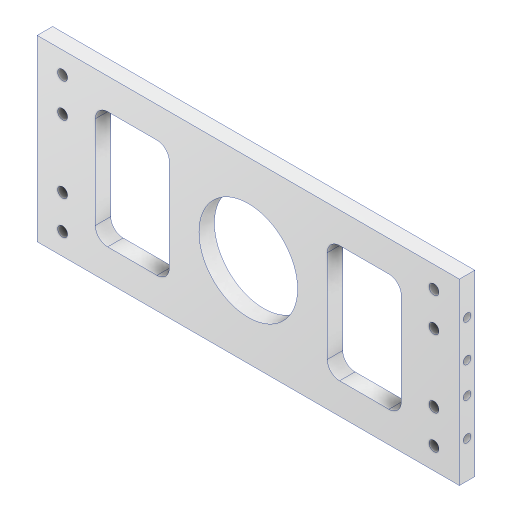
# Autodesk Inventor part: 조인트3_박스아랫판_6T
Saved by Autodesk Inventor 2023.2 (Build 272271000, 271)
## iProperties
Created: 2022-01-24
Part Number: 조인트3_박스아랫판_6T
Material: 알루미늄 6061
Document SubType Name: Modeling
Designer: BAEK
Density: 2.7 g/cm^3
Appearance: 알루미늄 - 평지
Mass: 60.1981 g
Surface Area: 152.316 cm^2
Volume: 22.2956 cm^3
Author: BAEK
Autodesk Inventor part; units mm, degrees
ref_plane "YZ Plane" through (0, 0, 0) normal (1, 0, 0) x (0, 1, 0)
ref_plane "XZ Plane" through (0, 0, 0) normal (0, 1, 0) x (-1, 0, 0)
ref_plane "XY Plane" through (0, 0, 0) normal (0, 0, 1) x (1, 0, 0)
sketch "스케치1" plane through (0, 0, 0) normal (0, 0, 1) x (1, 0, 0)
  line L0 (0, 0) -> (0, 58)
  line L1 (0, 58) -> (129.5, 58)
  line L2 (31.75, 58) -> (31.75, 0) construction
  circle A0 centre (31.75, 51) radius 1.6
  circle A1 centre (31.75, 40) radius 1.6
  circle A2 centre (31.75, 18) radius 1.6
  circle A3 centre (31.75, 7) radius 1.6
  line L3 (64.75, 58) -> (64.75, 0) construction
  circle A4 centre (97.75, 51) radius 1.6
  circle A5 centre (97.75, 40) radius 1.6
  circle A6 centre (97.75, 18) radius 1.6
  circle A7 centre (97.75, 7) radius 1.6
  line L4 (129.5, 58) -> (129.5, 0)
  line L5 (129.5, 0) -> (0, 0)
  circle A8 centre (64.75, 29) radius 10
  dimension "d0" = 58
  dimension "d1" = 129.5
  dimension "d3" = 3.2
  dimension "d4" = 3.2
  dimension "d5" = 3.2
  dimension "d6" = 3.2
  dimension "d7" = 7
  dimension "d8" = 11
  dimension "d9" = 7
  dimension "d10" = 11
  dimension "d13" = 66
  dimension "d14" = 20
  constraints: 12 end point, 9 centre point, 5 point on line, 4 symmetric about line, 4 vertical, 2 midpoint, 2 perpendicular, 4 other
  measures "d0" distance of L0.start L0.end
  measures "d1" distance of L0.end L1.end
  measures "d3" diameter of A0
  measures "d4" diameter of A1
  measures "d5" diameter of A2
  measures "d6" diameter of A3
  measures "d7" distance of L2.start A0.centre
  measures "d8" distance of A0.centre A1.centre
  measures "d9" distance of L2.end A3.centre
  measures "d10" distance of A2.centre A3.centre
  measures "d13" distance of A4.centre A0.centre
  measures "d14" diameter of A8
extrude "돌출1" add sketch "스케치1" along normal blind 4 contours L0 L1 L4 L5 | A8
extrude "돌출2" cut sketch "스케치1" along normal blind 4 contours A8
sketch "스케치2" plane through (0, 0, 4) normal (0, 0, 1) x (1, 0, 0)
  circle A0 centre (64.75, 29) radius 10 projected
  line L0 (0, 58) -> (0, 0) projected
  line L1 (0, 0) -> (129.5, 0) projected
  line L2 (129.5, 0) -> (129.5, 58) projected
  line L3 (129.5, 58) -> (0, 58) projected
  circle A1 centre (97.75, 7) radius 1.6 projected
  circle A2 centre (97.75, 18) radius 1.6 projected
  circle A3 centre (97.75, 40) radius 1.6 projected
  circle A4 centre (97.75, 51) radius 1.6 projected
  circle A5 centre (31.75, 7) radius 1.6 projected
  circle A6 centre (31.75, 18) radius 1.6 projected
  circle A7 centre (31.75, 40) radius 1.6 projected
  circle A8 centre (31.75, 51) radius 1.6 projected
  line L4 (41.75, 51) -> (87.75, 51)
  line L5 (89.75, 49) -> (89.75, 48)
  line L6 (87.75, 46) -> (41.75, 46)
  line L7 (39.75, 48) -> (39.75, 49)
  line L8 (0, 58) -> (0, 0) projected
  line L9 (0, 29) -> (129.5, 29) construction
  line L10 (41.75, 7) -> (87.75, 7)
  line L11 (89.75, 9) -> (89.75, 10)
  line L12 (87.75, 12) -> (41.75, 12)
  line L13 (39.75, 10) -> (39.75, 9)
  arc A9 (41.75, 51) -> (39.75, 49) centre (41.75, 49) ccw
  arc A10 (39.75, 48) -> (41.75, 46) centre (41.75, 48) ccw
  arc A11 (89.75, 49) -> (87.75, 51) centre (87.75, 49) ccw
  arc A12 (87.75, 46) -> (89.75, 48) centre (87.75, 48) ccw
  arc A13 (89.75, 10) -> (87.75, 12) centre (87.75, 10) ccw
  arc A14 (87.75, 7) -> (89.75, 9) centre (87.75, 9) ccw
  arc A15 (39.75, 9) -> (41.75, 7) centre (41.75, 9) ccw
  arc A16 (41.75, 12) -> (39.75, 10) centre (41.75, 10) ccw
  point P0 (39.75, 51)
  point P1 (89.75, 51)
  point P2 (89.75, 46)
  point P3 (39.75, 46)
  point P4 (39.75, 7)
  point P5 (89.75, 7)
  point P6 (89.75, 12)
  point P7 (39.75, 12)
  dimension "d17" = 50
  dimension "d18" = 5
  dimension "d19" = 8
  dimension "d22" = 2
  constraints: 18 end point, 16 point on circle, 16 point on line, 16 tangent, 8 centre point, 7 equal radius, 4 symmetric about line, 2 midpoint, 2 perpendicular, 1 horizontal, 1 vertical
  measures "d17" distance of point (39.75, 51) point (89.75, 51)
  measures "d18" distance of point (89.75, 51) point (89.75, 46)
  measures "d19" distance from line of A8.centre L7
  measures "d22" radius of A9
extrude "돌출3" cut sketch "스케치2" against normal blind 4 contours L4 A11 L5 A12 L6 A10 L7 A9 | A15 L13 A16 L12 A13 L11 A14 L10
sketch "스케치3" plane through (0, 0, 4) normal (0, 0, 1) x (1, 0, 0)
  line L0 (41.75, 12) -> (87.75, 12) projected
  arc A0 (89.75, 10) -> (87.75, 12) centre (87.75, 10) ccw projected
  line L1 (89.75, 10) -> (89.75, 9) projected
  arc A1 (87.75, 7) -> (89.75, 9) centre (87.75, 9) ccw projected
  line L2 (87.75, 7) -> (41.75, 7) projected
  arc A2 (39.75, 9) -> (41.75, 7) centre (41.75, 9) ccw projected
  line L3 (39.75, 9) -> (39.75, 10) projected
  arc A3 (41.75, 12) -> (39.75, 10) centre (41.75, 10) ccw projected
  arc A4 (87.75, 46) -> (89.75, 48) centre (87.75, 48) ccw projected
  line L4 (87.75, 46) -> (41.75, 46) projected
  arc A5 (39.75, 48) -> (41.75, 46) centre (41.75, 48) ccw projected
  line L5 (39.75, 48) -> (39.75, 49) projected
  arc A6 (41.75, 51) -> (39.75, 49) centre (41.75, 49) ccw projected
  line L6 (41.75, 51) -> (87.75, 51) projected
  arc A7 (89.75, 49) -> (87.75, 51) centre (87.75, 49) ccw projected
  line L7 (89.75, 49) -> (89.75, 48) projected
  circle A8 centre (64.75, 29) radius 10 projected
  line L8 (129.5, 0) -> (129.5, 58) projected
  line L9 (129.5, 58) -> (0, 58) projected
  line L10 (0, 58) -> (0, 0) projected
  line L11 (0, 0) -> (129.5, 0) projected
  circle A9 centre (97.75, 7) radius 1.6 projected
  circle A10 centre (97.75, 18) radius 1.6 projected
  circle A11 centre (97.75, 40) radius 1.6 projected
  circle A12 centre (97.75, 51) radius 1.6 projected
  circle A13 centre (31.75, 7) radius 1.6 projected
  circle A14 centre (31.75, 18) radius 1.6 projected
  circle A15 centre (31.75, 40) radius 1.6 projected
  circle A16 centre (31.75, 51) radius 1.6 projected
  line L12 (129.5, 58) -> (0, 58) projected
  line L13 (4.5, 58) -> (4.5, 0)
  line L14 (0, 0) -> (129.5, 0) projected
  circle A17 centre (4.5, 51) radius 1.6
  circle A18 centre (4.5, 40) radius 1.6
  circle A19 centre (4.5, 18) radius 1.6
  circle A20 centre (4.5, 7) radius 1.6
  line L15 (64.75, 58) -> (64.75, 0)
  circle A21 centre (125, 51) radius 1.6
  circle A22 centre (125, 40) radius 1.6
  circle A23 centre (125, 18) radius 1.6
  circle A24 centre (125, 7) radius 1.6
  dimension "d23" = 4.5
  dimension "d24" = 3.2
  dimension "d25" = 3.2
  dimension "d26" = 3.2
  dimension "d27" = 3.2
  constraints: 8 centre point, 6 point on line, 4 end point, 4 symmetric about line, 2 midpoint, 1 perpendicular, 4 other
  measures "d23" distance between parallel lines of L10 L13
  measures "d24" diameter of A17
  measures "d25" diameter of A18
  measures "d26" diameter of A19
  measures "d27" diameter of A20
extrude "돌출4" cut sketch "스케치3" against normal blind 4 contours A20 L13 | L13 A20 | A19 L13 | L13 A19 | A17 L13 | L13 A17 | A18 L13 | L13 A18 | A21 | A22 | A23 | A24
sketch "스케치5" plane through (0, 0, 4) normal (0, 0, 1) x (1, 0, 0)
  circle A0 centre (4.5, 18) radius 1.6 projected
  circle A1 centre (125, 18) radius 1.6 projected
  circle A2 centre (125, 40) radius 1.6 projected
  circle A3 centre (4.5, 40) radius 1.6 projected
  circle A4 centre (4.5, 7) radius 1.6 projected
  circle A5 centre (125, 7) radius 1.6 projected
  circle A6 centre (125, 51) radius 1.6 projected
  circle A7 centre (4.5, 51) radius 1.6 projected
  line L0 (41.75, 12) -> (87.75, 12) projected
  arc A8 (89.75, 10) -> (87.75, 12) centre (87.75, 10) ccw projected
  line L1 (89.75, 10) -> (89.75, 9) projected
  arc A9 (87.75, 7) -> (89.75, 9) centre (87.75, 9) ccw projected
  line L2 (87.75, 7) -> (41.75, 7) projected
  arc A10 (39.75, 9) -> (41.75, 7) centre (41.75, 9) ccw projected
  line L3 (39.75, 9) -> (39.75, 10) projected
  arc A11 (41.75, 12) -> (39.75, 10) centre (41.75, 10) ccw projected
  arc A12 (87.75, 46) -> (89.75, 48) centre (87.75, 48) ccw projected
  line L4 (87.75, 46) -> (41.75, 46) projected
  arc A13 (39.75, 48) -> (41.75, 46) centre (41.75, 48) ccw projected
  line L5 (39.75, 48) -> (39.75, 49) projected
  arc A14 (41.75, 51) -> (39.75, 49) centre (41.75, 49) ccw projected
  line L6 (41.75, 51) -> (87.75, 51) projected
  arc A15 (89.75, 49) -> (87.75, 51) centre (87.75, 49) ccw projected
  line L7 (89.75, 49) -> (89.75, 48) projected
  circle A16 centre (64.75, 29) radius 10 projected
  line L8 (129.5, 0) -> (129.5, 58) projected
  line L9 (129.5, 58) -> (0, 58) projected
  line L10 (0, 58) -> (0, 0) projected
  line L11 (0, 0) -> (129.5, 0) projected
  circle A17 centre (97.75, 7) radius 1.6 projected
  circle A18 centre (97.75, 51) radius 1.6 projected
  circle A19 centre (31.75, 7) radius 1.6 projected
  circle A20 centre (31.75, 51) radius 1.6 projected
  line L12 (129.5, 58) -> (0, 58) projected
  line L13 (64.75, 58) -> (-3.75, 58)
  line L14 (129.5, 58) -> (0, 58) projected
  line L15 (64.75, 58) -> (133.25, 58)
  line L16 (-3.75, 58) -> (-3.75, 0)
  line L17 (0, 0) -> (129.5, 0) projected
  line L18 (-3.75, 0) -> (0, 0)
  line L19 (133.25, 58) -> (133.25, 0)
  line L20 (133.25, 0) -> (129.5, 0)
  dimension "d36" = 68.5
  dimension "d37" = 68.5
  constraints: 12 end point, 2 perpendicular, 2 vertical, 1 horizontal, 1 midpoint, 1 point on line
  measures "d36" distance of L13.start L13.end
  measures "d37" distance of L13.start L15.end
extrude "돌출6" add sketch "스케치5" against normal up to surface (4 mm away) contours L8 L15 L19 L20 | L18 L16 L13 L10
sketch "스케치6" plane through (0, 0, 4) normal (0, 0, 1) x (1, 0, 0)
  circle A0 centre (4.5, 18) radius 1.6 projected
  circle A1 centre (125, 18) radius 1.6 projected
  circle A2 centre (125, 40) radius 1.6 projected
  circle A3 centre (4.5, 40) radius 1.6 projected
  circle A4 centre (4.5, 7) radius 1.6 projected
  circle A5 centre (125, 7) radius 1.6 projected
  circle A6 centre (125, 51) radius 1.6 projected
  circle A7 centre (4.5, 51) radius 1.6 projected
  line L0 (41.75, 12) -> (87.75, 12) projected
  arc A8 (89.75, 10) -> (87.75, 12) centre (87.75, 10) ccw projected
  line L1 (89.75, 10) -> (89.75, 9) projected
  arc A9 (87.75, 7) -> (89.75, 9) centre (87.75, 9) ccw projected
  line L2 (87.75, 7) -> (41.75, 7) projected
  arc A10 (39.75, 9) -> (41.75, 7) centre (41.75, 9) ccw projected
  line L3 (39.75, 9) -> (39.75, 10) projected
  arc A11 (41.75, 12) -> (39.75, 10) centre (41.75, 10) ccw projected
  arc A12 (87.75, 46) -> (89.75, 48) centre (87.75, 48) ccw projected
  line L4 (87.75, 46) -> (41.75, 46) projected
  arc A13 (39.75, 48) -> (41.75, 46) centre (41.75, 48) ccw projected
  line L5 (39.75, 48) -> (39.75, 49) projected
  arc A14 (41.75, 51) -> (39.75, 49) centre (41.75, 49) ccw projected
  line L6 (41.75, 51) -> (87.75, 51) projected
  arc A15 (89.75, 49) -> (87.75, 51) centre (87.75, 49) ccw projected
  line L7 (89.75, 49) -> (89.75, 48) projected
  circle A16 centre (64.75, 29) radius 10 projected
  line L8 (133.25, 58) -> (-3.75, 58) projected
  line L9 (-3.75, 58) -> (-3.75, 0) projected
  line L10 (-3.75, 0) -> (133.25, 0) projected
  line L11 (133.25, 0) -> (133.25, 58) projected
  circle A17 centre (97.75, 7) radius 1.6 projected
  circle A18 centre (97.75, 51) radius 1.6 projected
  circle A19 centre (31.75, 7) radius 1.6 projected
  circle A20 centre (31.75, 51) radius 1.6 projected
  point P0 (0, 0)
extrude "돌출7" add sketch "스케치6" along normal blind 1 contours L11 L10 L9 L8 | A17 | A18 | A19 | A20
sketch "스케치7" plane through (133.25, 0, 0) normal (1, 0, 0) x (0, 0, -1)
  line L0 (0, 58) -> (-5, 58) projected
  line L1 (-2.5, 58) -> (-2.5, 0) construction
  circle A0 centre (-2.5, 34) radius 1.25
  circle A1 centre (-2.5, 46) radius 1.25
  circle A2 centre (-2.5, 24) radius 1.25
  circle A3 centre (-2.5, 12) radius 1.25
  line L2 (0, 58) -> (-5, 58) projected
  line L3 (-5, 0) -> (0, 0) projected
  dimension "d43" = 12
  dimension "d46" = 12
  dimension "d49" = 12
  dimension "d50" = 12
  constraints: 4 centre point, 4 point on line, 3 midpoint, 2 end point, 2 equal radius, 1 vertical
  measures "d43" distance of A0.centre A1.centre
  measures "d46" distance of A2.centre A3.centre
  measures "d49" distance of point (-2.5, 58) A1.centre
  measures "d50" distance of point (-2.5, 0) A3.centre
extrude "돌출8" cut sketch "스케치7" against normal blind 10
sketch "스케치8" plane through (0, 0, 5) normal (0, 0, 1) x (1, 0, 0)
  line L0 (-3.75, 58) -> (-3.75, 0) projected
  line L1 (-3.75, 0) -> (133.25, 0) projected
  line L2 (133.25, 0) -> (133.25, 58) projected
  line L3 (133.25, 58) -> (-3.75, 58) projected
  circle A0 centre (64.75, 29) radius 10 projected
  circle A1 centre (4.5, 18) radius 1.6 projected
  circle A2 centre (125, 18) radius 1.6 projected
  circle A3 centre (125, 40) radius 1.6 projected
  circle A4 centre (4.5, 40) radius 1.6 projected
  circle A5 centre (4.5, 7) radius 1.6 projected
  circle A6 centre (125, 7) radius 1.6 projected
  circle A7 centre (125, 51) radius 1.6 projected
  circle A8 centre (4.5, 51) radius 1.6 projected
  line L4 (39.75, 48) -> (39.75, 49) projected
  arc A9 (41.75, 51) -> (39.75, 49) centre (41.75, 49) ccw projected
  line L5 (41.75, 51) -> (87.75, 51) projected
  arc A10 (89.75, 49) -> (87.75, 51) centre (87.75, 49) ccw projected
  line L6 (89.75, 49) -> (89.75, 48) projected
  arc A11 (87.75, 46) -> (89.75, 48) centre (87.75, 48) ccw projected
  line L7 (87.75, 46) -> (41.75, 46) projected
  arc A12 (39.75, 48) -> (41.75, 46) centre (41.75, 48) ccw projected
  line L8 (39.75, 9) -> (39.75, 10) projected
  arc A13 (41.75, 12) -> (39.75, 10) centre (41.75, 10) ccw projected
  line L9 (41.75, 12) -> (87.75, 12) projected
  arc A14 (89.75, 10) -> (87.75, 12) centre (87.75, 10) ccw projected
  line L10 (89.75, 10) -> (89.75, 9) projected
  arc A15 (87.75, 7) -> (89.75, 9) centre (87.75, 9) ccw projected
  line L11 (87.75, 7) -> (41.75, 7) projected
  arc A16 (39.75, 9) -> (41.75, 7) centre (41.75, 9) ccw projected
  point P0 (0, 0)
extrude "돌출9" add sketch "스케치8" against normal blind 5 contours L4 A9 L5 A10 L6 A11 L7 A12 | L8 A13 L9 A14 L10 A15 L11 A16
sketch "스케치9" plane through (0, 0, 5) normal (0, 0, 1) x (1, 0, 0)
  circle A0 centre (64.75, 29) radius 10 projected
  circle A1 centre (64.75, 29) radius 16
  line L0 (133.25, 58) -> (-3.75, 58) projected
  line L1 (35.75, 58) -> (64.75, 29)
  line L2 (64.75, 29) -> (70.75, 29)
  line L3 (-3.75, 0) -> (133.25, 0) projected
  line L4 (70.75, 29) -> (38.9302, 60.8198)
  point P0 (0, 0)
  point P1 (56.8413, 42.9087)
  point P2 (41.75, 58)
  point P3 (53.4363, 40.3137)
  dimension "d53" = 32
  dimension "d56" = 6
  dimension "d57" = 45
  dimension "d58" = 45
  constraints: 6 end point, 1 centre point, 1 coincident, 1 horizontal, 1 point on line
  measures "d53" diameter of A1
  measures "d56" distance of L1.end L2.end
  measures "d57" angle of L3 L1
  measures "d58" distance of L2.end L4.end
extrude "돌출10" cut sketch "스케치9" against normal blind 5 contours A0 L1 L2 L4 | A0 L4 A1 L1 | L4 L2 L1 A0 | A0 L1 A1 L4
sketch "스케치12" plane through (0, 0, 5) normal (0, 0, 1) x (1, 0, 0)
  line L0 (-3.75, 0) -> (-3.75, 58) projected
  line L1 (-3.75, 29) -> (133.25, 29) construction
  line L2 (133.25, 0) -> (133.25, 58) projected
  line L3 (19.111, 48) -> (35.111, 48)
  line L4 (39.111, 44) -> (39.111, 14)
  line L5 (35.111, 10) -> (19.111, 10)
  line L6 (15.111, 14) -> (15.111, 44)
  line L7 (15.111, 48) -> (39.111, 10) construction
  line L8 (39.111, 48) -> (15.111, 10) construction
  line L9 (133.25, 58) -> (-3.75, 58) projected
  arc A0 (19.111, 48) -> (15.111, 44) centre (19.111, 44) ccw
  arc A1 (39.111, 44) -> (35.111, 48) centre (35.111, 44) ccw
  arc A2 (35.111, 10) -> (39.111, 14) centre (35.111, 14) ccw
  arc A3 (15.111, 14) -> (19.111, 10) centre (19.111, 14) ccw
  line L10 (-3.75, 58) -> (133.25, 58) projected
  line L11 (64.75, 58) -> (64.75, 0)
  line L12 (133.25, 0) -> (-3.75, 0) projected
  line L13 (110.389, 48) -> (94.389, 48)
  line L14 (90.389, 44) -> (90.389, 14)
  line L15 (94.389, 10) -> (110.389, 10)
  line L16 (114.389, 14) -> (114.389, 44)
  line L17 (114.389, 48) -> (90.389, 10) construction
  line L18 (90.389, 48) -> (114.389, 10) construction
  arc A4 (114.389, 44) -> (110.389, 48) centre (110.389, 44) ccw
  arc A5 (94.389, 48) -> (90.389, 44) centre (94.389, 44) ccw
  arc A6 (90.389, 14) -> (94.389, 10) centre (94.389, 14) ccw
  arc A7 (110.389, 10) -> (114.389, 14) centre (110.389, 14) ccw
  point P0 (0, 0)
  point P1 (27.111, 29)
  point P2 (102.389, 29)
  dimension "d65" = 24
  dimension "d66" = 10
  dimension "d67" = 4
  constraints: 28 end point, 17 point on line, 17 symmetric about line, 16 point on circle, 8 centre point, 8 tangent, 6 midpoint, 3 equal radius, 2 parallel, 1 horizontal, 1 perpendicular, 4 other
  measures "d65" distance of L7.end L8.end
  measures "d66" distance between parallel lines of L9 L3
  measures "d67" radius of A0
extrude "돌출11" cut sketch "스케치12" against normal blind 5 contours L3 A1 L4 A2 L5 A3 L6 A0 | A4 L16 A7 L15 A6 L14 A5 L13
sketch "스케치13" plane through (97.75, 51, 4) normal (0, 0, -1) x (-1, 0, 0)
  arc A0 (3.361, -41) -> (7.361, -37) centre (3.361, -37) ccw projected
  line L0 (3.361, -41) -> (-12.639, -41) projected
  arc A1 (-16.639, -37) -> (-12.639, -41) centre (-12.639, -37) ccw projected
  line L1 (-16.639, -37) -> (-16.639, -7) projected
  arc A2 (-12.639, -3) -> (-16.639, -7) centre (-12.639, -7) ccw projected
  line L2 (-12.639, -3) -> (3.361, -3) projected
  arc A3 (7.361, -7) -> (3.361, -3) centre (3.361, -7) ccw projected
  line L3 (7.361, -7) -> (7.361, -37) projected
  arc A4 (58.639, -37) -> (62.639, -41) centre (62.639, -37) ccw projected
  line L4 (58.639, -37) -> (58.639, -7) projected
  arc A5 (62.639, -3) -> (58.639, -7) centre (62.639, -7) ccw projected
  line L5 (62.639, -3) -> (78.639, -3) projected
  arc A6 (82.639, -7) -> (78.639, -3) centre (78.639, -7) ccw projected
  line L6 (82.639, -7) -> (82.639, -37) projected
  arc A7 (78.639, -41) -> (82.639, -37) centre (78.639, -37) ccw projected
  line L7 (78.639, -41) -> (62.639, -41) projected
  circle A8 centre (33, -22) radius 16 projected
  circle A9 centre (93.25, -33) radius 1.6 projected
  circle A10 centre (-27.25, -33) radius 1.6 projected
  circle A11 centre (-27.25, -11) radius 1.6 projected
  circle A12 centre (93.25, -11) radius 1.6 projected
  circle A13 centre (93.25, -44) radius 1.6 projected
  circle A14 centre (-27.25, -44) radius 1.6 projected
  circle A15 centre (-27.25, 0) radius 1.6 projected
  circle A16 centre (93.25, 0) radius 1.6 projected
  line L8 (-35.5, -51) -> (101.5, -51) projected
  line L9 (101.5, -51) -> (101.5, 7) projected
  line L10 (101.5, 7) -> (-35.5, 7) projected
  line L11 (-35.5, 7) -> (-35.5, -51) projected
  circle A17 centre (0, -44) radius 1.6 projected
  circle A18 centre (0, 0) radius 1.6 projected
  circle A19 centre (66, -44) radius 1.6 projected
  circle A20 centre (66, 0) radius 1.6 projected
  point P0 (97.75, -51)
extrude "돌출12" add sketch "스케치13" along normal up to surface (4 mm away) contours A17 | A18 | A19 | A20
sketch "스케치14" plane through (-3.75, 0, 0) normal (-1, 0, 0) x (0, 0, 1)
  line L0 (0, 58) -> (5, 58) projected
  line L1 (2.5, 58) -> (2.5, 0) construction
  line L2 (5, 0) -> (0, 0) projected
  circle A0 centre (2.5, 46) radius 1.25 projected
  circle A1 centre (2.5, 34) radius 1.25 projected
  circle A2 centre (2.5, 24) radius 1.25 projected
  circle A3 centre (2.5, 12) radius 1.25 projected
  constraints: 2 end point, 2 midpoint
extrude "돌출13" cut sketch "스케치14" against normal blind 10
